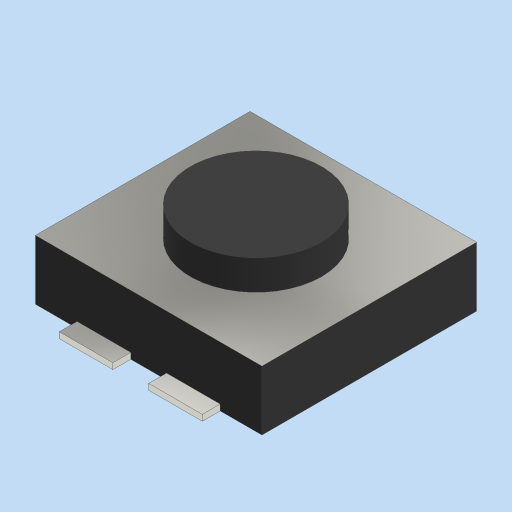
# Autodesk Inventor part: R-667842_tactile_switch
Saved by Autodesk Inventor 2024 (Build 280153000, 153)
## iProperties
Created: 2025-05-11
Part Number: R-667842_tactile_switch
Material: Generic
Document SubType Name: Modeling
Designer: XxPan
Density: 1 g/cm^3
Appearance: Default
Author: XxPan
Autodesk Inventor part; units mm, degrees
ref_plane "YZ Plane" through (0, 0, 0) normal (1, 0, 0) x (0, 1, 0)
ref_plane "XZ Plane" through (0, 0, 0) normal (0, 1, 0) x (-1, 0, 0)
ref_plane "XY Plane" through (0, 0, 0) normal (0, 0, 1) x (1, 0, 0)
sketch "Sketch1" plane through (0, 0, 0) normal (0, 1, 0) x (-1, 0, 0)
  line L0 (1.9, 1.8) -> (-1.9, 1.8)
  line L1 (-1.9, 1.8) -> (-1.9, -1.8)
  line L2 (-1.9, -1.8) -> (1.9, -1.8)
  line L3 (1.9, -1.8) -> (1.9, 1.8)
  line L4 (2.66, 0) -> (-2.66, 0) construction
  line L5 (0, -2.52) -> (0, 2.52) construction
  point P0 (0, 0)
  dimension "d0" = 3.8
  dimension "d1" = 3.6
  constraints: 8 end point, 2 parallel, 1 horizontal, 1 perpendicular, 2 other
  measures "d0" distance of L2.end L1.end
  measures "d1" distance of L1.end L0.end
extrude "Extrusion1" add sketch "Sketch1" along normal blind 1
sketch "Sketch2" plane through (0, 1, 0) normal (0, 1, 0) x (1, 0, 0)
  circle A0 centre (0, 0) radius 1.1
  dimension "d4" = 2.2
  constraints: 1 centre point, 1 coincident
  measures "d4" diameter of A0
extrude "Extrusion2" add sketch "Sketch2" along normal blind 0.5
sketch "Sketch3" plane through (0, 0, 0) normal (0, -1, 0) x (1, 0, 0)
  line L0 (1.2, -1.6) -> (0.3, -1.6)
  line L1 (0.3, -1.6) -> (0.3, -2.1)
  line L2 (0.3, -2.1) -> (1.2, -2.1)
  line L3 (1.2, -2.1) -> (1.2, -1.6)
  line L4 (-0.3, -1.6) -> (-1.2, -1.6)
  line L5 (-1.2, -1.6) -> (-1.2, -2.1)
  line L6 (-1.2, -2.1) -> (-0.3, -2.1)
  line L7 (-0.3, -2.1) -> (-0.3, -1.6)
  line L8 (1.2, 2.1) -> (0.3, 2.1)
  line L9 (0.3, 2.1) -> (0.3, 1.6)
  line L10 (0.3, 1.6) -> (1.2, 1.6)
  line L11 (1.2, 1.6) -> (1.2, 2.1)
  line L12 (-0.3, 2.1) -> (-1.2, 2.1)
  line L13 (-1.2, 2.1) -> (-1.2, 1.6)
  line L14 (-1.2, 1.6) -> (-0.3, 1.6)
  line L15 (-0.3, 1.6) -> (-0.3, 2.1)
  point P0 (0, 0)
  dimension "d7" = 3.2
  dimension "d8" = 4.2
  dimension "d9" = 0.5
  dimension "d10" = 0.6
  dimension "d11" = 2.4
  dimension "d12" = 1.6
  dimension "d13" = 0.3
  constraints: 32 end point, 8 parallel, 6 collinear, 4 horizontal, 4 perpendicular, 3 point on line
  measures "d7" distance between parallel lines of L0 L10
  measures "d8" distance between parallel lines of L2 L8
  measures "d9" distance of L2.end L0.start
  measures "d10" distance between parallel lines of L7 L1
  measures "d11" distance between parallel lines of L3 L5
  measures "d12" distance from line of point (0, 0) L0
  measures "d13" distance from line of point (0, 0) L1
extrude "Extrusion3" add sketch "Sketch3" against normal blind 0.1
equation "\"d9\" = -0.5 * d7 + 0.5 * d8"
equation "\"d12\" = 0.5 * d7"
equation "\"d13\" = 0.5 * d10"
body "Solid1"
